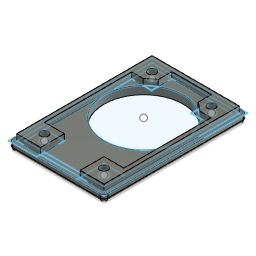
Case-MQ2-Top_v4 (Autodesk Fusion 360 design; units mm, degrees)
Autodesk Fusion 360 part; units mm, degrees
sketch "Sketch1" plane through (0, 0, 0) normal (0, 1, 0) x (1, 0, 0)
  line L0 (-10, -10) -> (10, -10)
  line L1 (10, -10) -> (10, 22.1)
  line L2 (10, 22.1) -> (-10, 22.1)
  line L3 (-10, 22.1) -> (-10, -10)
  line L4 (-12, -12) -> (12, -12)
  line L5 (12, -12) -> (12, 24.1)
  line L6 (12, 24.1) -> (-12, 24.1)
  line L7 (-12, 24.1) -> (-12, -12)
  circle A0 centre (0, 10) radius 10
  line L8 (5, -10) -> (5, -12)
  line L9 (-5, -10) -> (-5, -12)
  line L10 (-5, -10) -> (-5, -5)
  line L11 (-5, -5) -> (-10, -5)
  line L12 (5, -10) -> (5, -5)
  line L13 (5, -5) -> (10, -5)
  line L14 (-5, -11) -> (-11, -11)
  line L15 (-11, -11) -> (-11, 23.1)
  line L16 (-11, 23.1) -> (11, 23.1)
  line L17 (11, 23.1) -> (11, -11)
  line L18 (11, -11) -> (5, -11)
  line L19 (-5, -11) -> (5, -11)
  line L20 (-10, 17) -> (-7.1414, 17)
  line L21 (-7.1414, 17) -> (-5, 17)
  line L22 (-5, 17) -> (-5, 18.6603)
  line L23 (-5, 18.6603) -> (-5, 22.1)
  line L24 (10, 17) -> (7.1414, 17)
  line L25 (5, 17) -> (5, 18.6603)
  line L26 (5, 22.1) -> (5, 18.6603)
  line L27 (5, 17) -> (7.1414, 17)
  circle A1 centre (-7.5, -7.5) radius 1
  circle A2 centre (7.5, -7.5) radius 1
  circle A3 centre (-7.5, 19.6) radius 1
  circle A4 centre (7.5, 19.6) radius 1
  dimension "d1" = 32.1
  dimension "d2" = 36.1
  dimension "d3" = 34.1
  dimension "d4" = 2.5
  dimension "d5" = 2.5
  dimension "d6" = 2.5
  dimension "d7" = 2.5
  dimension "d8" = 2.5
  dimension "d9" = 2.5
  dimension "d10" = 2.5
  dimension "d11" = 2.5
  constraint horizontal L0
  constraint vertical L1
  constraint horizontal L2
  constraint vertical L3
  constraint horizontal L4
  constraint vertical L5
  constraint horizontal L6
  constraint vertical L7
  constraint tangent L3 A0
  constraint coincident L0 L8.start
  constraint coincident L4 L8.end
  constraint perpendicular L4 L8
  constraint coincident L0 L9.start
  constraint coincident L4 L9.end
  constraint perpendicular L4 L9
  constraint perpendicular L0 L10
  constraint coincident L3 L11.end
  constraint perpendicular L3 L11
  constraint perpendicular L0 L12
  constraint coincident L1 L13.end
  constraint perpendicular L1 L13
  constraint midpoint L9 L14.start
  constraint perpendicular L9 L14
  constraint perpendicular L15 L16
  constraint perpendicular L16 L17
  constraint midpoint L8 L18.end
  constraint perpendicular L8 L18
  constraint coincident L3 L20.start
  constraint coincident A0 L20.end
  constraint perpendicular L3 L20
  constraint perpendicular L3 L21
  constraint coincident A0 L22.end
  constraint perpendicular L21 L22
  constraint coincident L2 L23.end
  constraint perpendicular L2 L23
  constraint coincident L1 L24.start
  constraint coincident A0 L24.end
  constraint perpendicular L1 L24
  constraint coincident A0 L25.end
  constraint perpendicular L24 L25
  constraint coincident L2 L26.start
  constraint perpendicular L2 L26
  constraint perpendicular L25 L27
  measures "d1" distance of L0.start L2.end
  measures "d2" distance of L4.start L6.end
  measures "d3" distance of L14.end L15.end
  measures "d4" distance of L0 A1.centre
  measures "d5" distance of L3 A1.centre
  measures "d6" distance of L0 A2.centre
  measures "d7" distance of L1 A2.centre
  measures "d8" distance of L3 A3.centre
  measures "d9" distance of L2 A3.centre
  measures "d10" distance of L1 A4.centre
  measures "d11" distance of L2 A4.centre
extrude "Extrude1" add sketch "Sketch1" against normal blind 2 contours L0 L3 L10 L11 | L0 L1 L2 L3 L8 L9 L14 L15 L16 L17 L18 | L0 L1 L3 A0 L10 L11 L12 L13 | L0 L8 L9 L19 | L0 L1 L12 L13 | L4 L8 L9 L19 | L4 L5 L6 L7 L8 L9 L14 L15 L16 L17 L18 | L3 A0 L20 | A0 L21 L22 L25 L27 | L2 L3 A0 L20 L23 | A0 L21 L22 | L1 A0 L24 | L2 A0 L23 L26 | L1 L2 A0 L24 L26 | A0 L25 L27 | A1 | A2 | A3 | A4
extrude "Extrude2" add sketch "Sketch1" along normal blind 1.55 contours L0 L3 L10 L11 | L0 L1 L2 L3 L8 L9 L14 L15 L16 L17 L18 | L0 L1 L12 L13 | L2 L3 A0 L20 L23 | L1 L2 A0 L24 L26
extrude "Extrude3" cut sketch "Sketch1" against normal blind 4 contours A0 L21 L22 L25 L27 | A0 L21 L22 | A0 L25 L27 | A1 | A2 | A3 | A4
fillet "Fillet1" radius 1 4 edges at (-12, -2, -6.05) (0, -2, 12) (12, -2, -6.05) (0, -2, -24.1)
fillet "Fillet2" radius 1 8 edges at (12, -0.5, 12) (11.7071, -1.7071, 11.7071) (-12, -0.5, 12) (-11.7071, -1.7071, 11.7071) (-12, -0.5, -24.1) (-11.7071, -1.7071, -23.8071) (12, -0.5, -24.1) (11.7071, -1.7071, -23.8071)
